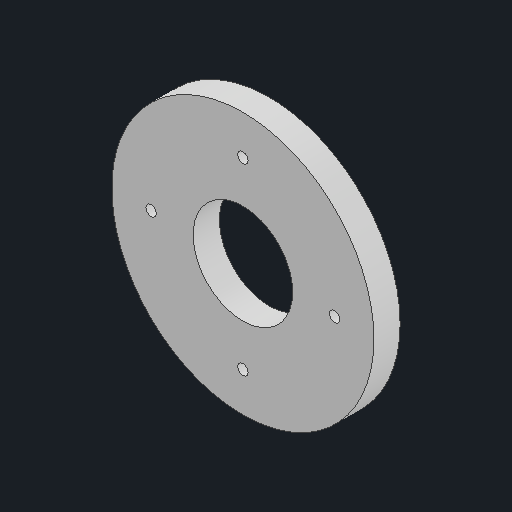
# Autodesk Inventor part: drive sprocket flange
Saved by Autodesk Inventor 2023.2 (Build 272271030, 271C)
## iProperties
Created: 2023-04-05
Part Number: drive sprocket flange
Material: Generic
Document SubType Name: Modeling
Designer: ralph
Density: 1 g/cm^3
Appearance: Default
Author: ralph
Autodesk Inventor part; units mm, degrees
ref_plane "YZ Plane" through (0, 0, 0) normal (1, 0, 0) x (0, 1, 0)
ref_plane "XZ Plane" through (0, 0, 0) normal (0, 1, 0) x (-1, 0, 0)
ref_plane "XY Plane" through (0, 0, 0) normal (0, 0, 1) x (1, 0, 0)
sketch "Sketch1" plane through (0, 0, 0) normal (0, 0, 1) x (1, 0, 0)
  arc A0 (9.4191, 43.3754) -> (11.0761, 45.5644) centre (1.4765, 51.109) ccw projected
  arc A1 (2.6827, 44.1627) -> (9.4191, 43.3754) centre (6.35, 46.3277) ccw projected
  arc A2 (1.5753, 46.6749) -> (2.6827, 44.1627) centre (12.1948, 49.8562) ccw projected
  arc A3 (-9.4191, 43.3754) -> (-2.6827, 44.1627) centre (-6.35, 46.3277) ccw projected
  arc A4 (-11.0761, 45.5644) -> (-9.4191, 43.3754) centre (-1.4765, 51.109) ccw projected
  arc A5 (-21.0132, 39.8183) -> (-14.64, 42.138) centre (-18.7077, 43.3989) ccw projected
  arc A6 (-23.1303, 41.5662) -> (-21.0132, 39.8183) centre (-15.0682, 49.1752) ccw projected
  arc A7 (-31.4745, 33.6834) -> (-25.808, 37.4103) centre (-30.0568, 37.6992) ccw projected
  arc A8 (-33.9376, 34.896) -> (-31.4745, 33.6834) centre (-27.8475, 44.1591) ccw projected
  arc A9 (-40.2389, 25.3013) -> (-35.5847, 30.2346) centre (-39.7856, 29.5357) ccw projected
  arc A10 (-42.9153, 25.9131) -> (-40.2389, 25.3013) centre (-39.1256, 36.331) ccw projected
  arc A11 (-46.8341, 15.1239) -> (-43.443, 20.9975) centre (-47.3695, 19.3488) ccw projected
  arc A12 (-49.5794, 15.1021) -> (-46.8341, 15.1239) centre (-48.2944, 26.1131) ccw projected
  arc A13 (-50.9044, 3.6999) -> (-48.9593, 10.1973) centre (-52.3997, 7.6874) ccw projected
  arc A14 (-53.5707, 3.0455) -> (-50.9044, 3.6999) centre (-54.8597, 14.0561) ccw projected
  arc A15 (-52.2305, -8.3548) -> (-51.8361, -1.584) centre (-54.605, -4.8196) ccw projected
  arc A16 (-54.674, -9.6064) -> (-52.2305, -8.3548) centre (-58.4674, 0.8101) ccw projected
  arc A17 (-50.7408, -20.3904) -> (-51.9185, -13.7112) centre (-53.8666, -17.4981) ccw projected
  arc A18 (-52.8298, -22.1718) -> (-50.7408, -20.3904) centre (-58.9232, -12.9109) ccw projected
  arc A19 (-46.5156, -31.7581) -> (-49.2019, -25.5305) centre (-50.2242, -29.6646) ccw projected
  arc A20 (-48.1375, -33.9732) -> (-46.5156, -31.7581) centre (-56.2023, -26.3671) ccw projected
  arc A21 (-39.7828, -41.8449) -> (-43.8329, -36.4047) centre (-43.8742, -40.6631) ccw projected
  arc A22 (-40.8501, -44.3744) -> (-39.7828, -41.8449) centre (-50.4517, -38.8332) ccw projected
  arc A23 (-30.9053, -50.1072) -> (-36.1008, -45.7476) centre (-35.1589, -49.9008) ccw projected
  arc A24 (-31.3605, -52.8146) -> (-30.9053, -50.1072) centre (-41.9811, -49.637) ccw projected
  arc A25 (-20.3617, -56.0994) -> (-26.4225, -53.0555) centre (-24.5482, -56.8795) ccw projected
  arc A26 (-20.1802, -58.8388) -> (-20.3617, -56.0994) centre (-31.2473, -58.1962) ccw projected
  arc A27 (-8.7203, -59.4986) -> (-15.3198, -57.9345) centre (-12.6141, -61.2232) ccw projected
  arc A28 (-7.912, -62.1223) -> (-8.7203, -59.4986) centre (-18.829, -64.0493) ccw projected
  arc A29 (3.3911, -60.1215) -> (-3.3911, -60.1215) centre (0, -62.6976) ccw projected
  arc A30 (4.7827, -62.4881) -> (3.3911, -60.1215) centre (-5.3956, -66.8807) ccw projected
  arc A31 (15.3198, -57.9345) -> (8.7203, -59.4986) centre (12.6141, -61.2232) ccw projected
  arc A32 (17.2196, -59.9164) -> (15.3198, -57.9345) centre (8.3287, -66.5379) ccw projected
  arc A33 (26.4225, -53.0555) -> (20.3617, -56.0994) centre (24.5482, -56.8795) ccw projected
  arc A34 (28.7282, -54.5458) -> (26.4225, -53.0555) centre (21.6039, -63.0393) ccw projected
  arc A35 (36.1008, -45.7476) -> (30.9053, -50.1072) centre (35.1589, -49.9008) ccw projected
  arc A36 (38.688, -46.666) -> (36.1008, -45.7476) centre (33.7145, -56.5735) ccw projected
  arc A37 (43.8329, -36.4047) -> (39.7828, -41.8449) centre (43.8742, -40.6631) ccw projected
  arc A38 (46.5622, -36.7017) -> (43.8329, -36.4047) centre (44.0076, -47.4891) ccw projected
  arc A39 (49.2019, -25.5305) -> (46.5156, -31.7581) centre (50.2242, -29.6646) ccw projected
  arc A40 (51.9262, -25.19) -> (49.2019, -25.5305) centre (51.9282, -36.2758) ccw projected
  arc A41 (51.9185, -13.7112) -> (50.7408, -20.3904) centre (53.8666, -17.4981) ccw projected
  arc A42 (54.4908, -12.7517) -> (51.9185, -13.7112) centre (57.0493, -23.5382) ccw projected
  arc A43 (51.8361, -1.584) -> (52.2305, -8.3548) centre (54.605, -4.8196) ccw projected
  arc A44 (54.1178, -0.0572) -> (51.8361, -1.584) centre (59.0949, -9.9629) ccw projected
  arc A45 (48.9593, 10.1973) -> (50.9044, 3.6999) centre (52.3997, 7.6874) ccw projected
  arc A46 (50.8273, 12.2092) -> (48.9593, 10.1973) centre (57.9546, 3.7182) ccw projected
  arc A47 (43.443, 20.9975) -> (46.8341, 15.1239) centre (47.3695, 19.3488) ccw projected
  arc A48 (44.7967, 23.386) -> (43.443, 20.9975) centre (53.69, 16.7676) ccw projected
  arc A49 (35.5847, 30.2346) -> (40.2389, 25.3013) centre (39.7856, 29.5357) ccw projected
  arc A50 (36.3511, 32.8708) -> (35.5847, 30.2346) centre (46.531, 28.4818) ccw projected
  arc A51 (25.808, 37.4103) -> (31.4745, 33.6834) centre (30.0568, 37.6992) ccw projected
  arc A52 (25.9458, 40.1523) -> (25.808, 37.4103) centre (36.8635, 38.2292) ccw projected
  arc A53 (14.64, 42.138) -> (21.0132, 39.8183) centre (18.7077, 43.3989) ccw projected
  arc A54 (14.1417, 44.8378) -> (14.64, 42.138) centre (25.2086, 45.4844) ccw projected
  circle A55 centre (0, -8) radius 12.065
  circle A56 centre (0, -8) radius 22.225
  circle A57 centre (0, -8) radius 31.75
  circle A58 centre (22.225, -8) radius 1.27
  circle A59 centre (0, -30.225) radius 1.27
  circle A60 centre (-22.225, -8) radius 1.27
  circle A61 centre (0, 14.225) radius 1.27
  circle A62 centre (0, -8) radius 12.065 projected
  ellipse E0 centre (12.8803, 49.8016) end of major axis (24.6386, 49.2708) minor radius 11.3649 (1.4863, 46.9888) -> (1.5753, 46.6749) ccw projected
  line L0 (1.4863, 46.9888) -> (1.1981, 48.0928) projected
  arc A63 (1.1981, 48.0928) -> (0.2767, 50.1653) centre (-5.564, 46.3277) ccw projected
  arc A64 (0.2767, 50.1653) -> (-0.2767, 50.1653) centre (0, -8) ccw projected
  arc A65 (-0.2767, 50.1653) -> (-1.1981, 48.0928) centre (5.564, 46.3277) ccw projected
  line L1 (-1.1981, 48.0928) -> (-1.4863, 46.9888) projected
  arc A66 (-2.6827, 44.1627) -> (-1.5753, 46.6749) centre (-12.1948, 49.8562) ccw projected
  ellipse E1 centre (-0.7968, 51.214) end of major axis (10.7669, 53.4091) minor radius 11.3649 (-11.2351, 45.8493) -> (-11.0761, 45.5644) ccw projected
  line L2 (-11.2351, 45.8493) -> (-11.7701, 46.8571) projected
  arc A67 (-11.7701, 46.8571) -> (-13.1446, 48.6613) centre (-17.9429, 43.5802) ccw projected
  arc A68 (-13.1446, 48.6613) -> (-13.6831, 48.5337) centre (0, -8) ccw projected
  arc A69 (-13.6831, 48.5337) -> (-14.1017, 46.3046) centre (-7.1148, 46.1465) ccw projected
  line L3 (-14.1017, 46.3046) -> (-14.1275, 45.1638) projected
  arc A70 (-14.64, 42.138) -> (-14.1417, 44.8378) centre (-25.2086, 45.4844) ccw projected
  ellipse E2 centre (-14.431, 49.4341) end of major axis (-3.6852, 54.2369) minor radius 11.3649 (-23.3508, 41.8068) -> (-23.1303, 41.5662) ccw projected
  line L4 (-23.3508, 41.8068) -> (-24.1038, 42.6641) projected
  arc A71 (-24.1038, 42.6641) -> (-25.8573, 44.1026) centre (-29.3544, 38.0519) ccw projected
  arc A72 (-25.8573, 44.1026) -> (-26.3518, 43.8543) centre (0, -8) ccw projected
  arc A73 (-26.3518, 43.8543) -> (-26.2451, 41.5887) centre (-19.4101, 43.0461) ccw projected
  line L5 (-26.2451, 41.5887) -> (-26.0071, 40.4728) projected
  arc A74 (-25.808, 37.4103) -> (-25.9458, 40.1523) centre (-36.8635, 38.2292) ccw projected
  ellipse E3 centre (-27.2872, 44.5579) end of major axis (-17.9387, 51.7094) minor radius 11.3649 (-34.2076, 35.0792) -> (-33.9376, 34.896) ccw projected
  line L6 (-34.2076, 35.0792) -> (-35.138, 35.7397) projected
  arc A75 (-35.138, 35.7397) -> (-37.176, 36.7351) centre (-39.1835, 30.041) ccw projected
  arc A76 (-37.176, 36.7351) -> (-37.5999, 36.3794) centre (0, -8) ccw projected
  arc A77 (-37.5999, 36.3794) -> (-36.9736, 34.1995) centre (-30.6589, 37.1939) ccw projected
  line L7 (-36.9736, 34.1995) -> (-36.4847, 33.1685) projected
  arc A78 (-35.5847, 30.2346) -> (-36.3511, 32.8708) centre (-46.531, 28.4818) ccw projected
  ellipse E4 centre (-38.6724, 36.8483) end of major axis (-31.2251, 45.963) minor radius 11.3649 (-43.2203, 26.0292) -> (-42.9153, 25.9131) ccw projected
  line L8 (-43.2203, 26.0292) -> (-44.2779, 26.4573) projected
  arc A79 (-44.2779, 26.4573) -> (-46.4905, 26.9559) centre (-46.9001, 19.9793) ccw projected
  arc A80 (-46.4905, 26.9559) -> (-46.821, 26.512) centre (0, -8) ccw projected
  arc A81 (-46.821, 26.512) -> (-45.7088, 24.5353) centre (-40.2549, 28.9053) ccw projected
  line L9 (-45.7088, 24.5353) -> (-44.9953, 23.6449) projected
  arc A82 (-43.443, 20.9975) -> (-44.7967, 23.386) centre (-53.69, 16.7676) ccw projected
  ellipse E5 centre (-47.9727, 26.721) end of major axis (-42.8281, 37.3074) minor radius 11.3649 (-49.9029, 15.1447) -> (-49.5794, 15.1021) ccw projected
  line L10 (-49.9029, 15.1447) -> (-51.0308, 15.3173) projected
  arc A83 (-51.0308, 15.3173) -> (-53.2988, 15.2922) centre (-52.0884, 8.4092) ccw projected
  arc A84 (-53.2988, 15.2922) -> (-53.518, 14.784) centre (0, -8) ccw projected
  arc A85 (-53.518, 14.784) -> (-51.9799, 13.1172) centre (-47.6808, 18.6271) ccw projected
  line L11 (-51.9799, 13.1172) -> (-51.0803, 12.4152) projected
  arc A86 (-48.9593, 10.1973) -> (-50.8273, 12.2092) centre (-57.9546, 3.7182) ccw projected
  ellipse E6 centre (-54.6868, 14.7218) end of major axis (-52.1223, 26.2093) minor radius 11.3649 (-53.8953, 3.0124) -> (-53.5707, 3.0455) ccw projected
  line L12 (-53.8953, 3.0124) -> (-55.0326, 2.9203) projected
  arc A87 (-55.0326, 2.9203) -> (-57.2336, 2.3728) centre (-54.4685, -4.0456) ccw projected
  arc A88 (-57.2336, 2.3728) -> (-57.3297, 1.8278) centre (0, -8) ccw projected
  arc A89 (-57.3297, 1.8278) -> (-55.4487, 0.5606) centre (-52.5362, 6.9134) ccw projected
  line L13 (-55.4487, 0.5606) -> (-54.4115, 0.085) projected
  arc A90 (-51.8361, -1.584) -> (-54.1178, -0.0572) centre (-59.0949, -9.9629) ccw projected
  ellipse E7 centre (-58.4527, 1.4977) end of major axis (-58.6065, 13.2669) minor radius 11.3649 (-54.9822, -9.7136) -> (-54.674, -9.6064) ccw projected
  line L14 (-54.9822, -9.7136) -> (-56.0676, -10.0655) projected
  arc A91 (-56.0676, -10.0655) -> (-58.083, -11.1058) centre (-53.9123, -16.7135) ccw projected
  arc A92 (-58.083, -11.1058) -> (-58.0508, -11.6583) centre (0, -8) ccw projected
  arc A93 (-58.0508, -11.6583) -> (-55.9283, -12.4575) centre (-54.5593, -5.6043) ccw projected
  line L15 (-55.9283, -12.4575) -> (-54.8093, -12.6811) projected
  arc A94 (-51.9185, -13.7112) -> (-54.4908, -12.7517) centre (-57.0493, -23.5382) ccw projected
  ellipse E8 centre (-59.0674, -12.2385) end of major axis (-61.9313, -0.8219) minor radius 11.3649 (-53.105, -22.3471) -> (-52.8298, -22.1718) ccw projected
  line L16 (-53.105, -22.3471) -> (-54.08, -22.9399) projected
  arc A95 (-54.08, -22.9399) -> (-55.8011, -24.4169) centre (-50.4496, -28.9116) ccw projected
  arc A96 (-55.8011, -24.4169) -> (-55.6424, -24.9471) centre (0, -8) ccw projected
  arc A97 (-55.6424, -24.9471) -> (-53.3927, -25.2353) centre (-53.6412, -18.2511) ccw projected
  line L17 (-53.3927, -25.2353) -> (-52.2524, -25.1948) projected
  arc A98 (-49.2019, -25.5305) -> (-51.9262, -25.19) centre (-51.9282, -36.2758) ccw projected
  ellipse E9 centre (-56.4978, -25.7461) end of major axis (-61.9173, -15.2977) minor radius 11.3649 (-48.3648, -34.2073) -> (-48.1375, -33.9732) ccw projected
  line L18 (-48.3648, -34.2073) -> (-49.1769, -35.0089) projected
  arc A99 (-49.1769, -35.0089) -> (-50.511, -36.843) centre (-44.2672, -39.9824) ccw projected
  arc A100 (-50.511, -36.843) -> (-50.2343, -37.3223) centre (0, -8) ccw projected
  arc A101 (-50.2343, -37.3223) -> (-47.9788, -37.084) centre (-49.8312, -30.3453) ccw projected
  line L19 (-47.9788, -37.084) -> (-46.8786, -36.7815) projected
  arc A102 (-43.8329, -36.4047) -> (-46.5622, -36.7017) centre (-44.0076, -47.4891) ccw projected
  ellipse E10 centre (-50.8824, -38.297) end of major axis (-58.5653, -29.3801) minor radius 11.3649 (-41.0173, -44.6545) -> (-40.8501, -44.3744) ccw projected
  line L20 (-41.0173, -44.6545) -> (-41.6226, -45.6218) projected
  arc A103 (-41.6226, -45.6218) -> (-42.4978, -47.7142) centre (-35.6983, -49.3291) ccw projected
  arc A104 (-42.4978, -47.7142) -> (-42.118, -48.1167) centre (0, -8) ccw projected
  arc A105 (-42.118, -48.1167) -> (-39.9783, -47.3647) centre (-43.3348, -41.2348) ccw projected
  line L21 (-39.9783, -47.3647) -> (-38.9775, -46.8167) projected
  arc A106 (-36.1008, -45.7476) -> (-38.688, -46.666) centre (-33.7145, -56.5735) ccw projected
  ellipse E11 centre (-42.5239, -49.2147) end of major axis (-52.0561, -42.3099) minor radius 11.3649 (-31.4586, -53.1258) -> (-31.3605, -52.8146) ccw projected
  line L22 (-31.4586, -53.1258) -> (-31.8245, -54.2065) projected
  arc A107 (-31.8245, -54.2065) -> (-32.1936, -56.4444) centre (-25.2049, -56.4476) ccw projected
  arc A108 (-32.1936, -56.4444) -> (-31.7312, -56.7485) centre (0, -8) ccw projected
  arc A109 (-31.7312, -56.7485) -> (-29.8226, -55.5232) centre (-34.5022, -50.3327) ccw projected
  line L23 (-29.8226, -55.5232) -> (-28.9751, -54.7592) projected
  arc A110 (-26.4225, -53.0555) -> (-28.7282, -54.5458) centre (-21.6039, -63.0393) ccw projected
  ellipse E12 centre (-31.8729, -57.9104) end of major axis (-42.7405, -53.3901) minor radius 11.3649 (-20.2039, -59.1642) -> (-20.1802, -58.8388) ccw projected
  line L24 (-20.2039, -59.1642) -> (-20.3107, -60.3003) projected
  arc A111 (-20.3107, -60.3003) -> (-20.1537, -62.5629) centre (-13.3527, -60.9544) ccw projected
  arc A112 (-20.1537, -62.5629) -> (-19.6337, -62.7522) centre (0, -8) ccw projected
  arc A113 (-19.6337, -62.7522) -> (-18.0591, -61.1198) centre (-23.8096, -57.1484) ccw projected
  line L25 (-18.0591, -61.1198) -> (-17.4107, -60.1809) projected
  arc A114 (-15.3198, -57.9345) -> (-17.2196, -59.9164) centre (-8.3287, -66.5379) ccw projected
  ellipse E13 centre (-19.5036, -63.9154) end of major axis (-31.1208, -62.0232) minor radius 11.3649 (-7.86, -62.4444) -> (-7.912, -62.1223) ccw projected
  line L26 (-7.86, -62.4444) -> (-7.7019, -63.5745) projected
  arc A115 (-7.7019, -63.5745) -> (-7.0274, -65.7399) centre (-0.7807, -62.6063) ccw projected
  arc A116 (-7.0274, -65.7399) -> (-6.4777, -65.8042) centre (0, -8) ccw projected
  arc A117 (-6.4777, -65.8042) -> (-5.322, -63.8527) centre (-11.8334, -61.3144) ccw projected
  line L27 (-5.322, -63.8527) -> (-4.9076, -62.7895) projected
  arc A118 (-3.3911, -60.1215) -> (-4.7827, -62.4881) centre (5.3956, -66.8807) ccw projected
  ellipse E14 centre (-6.0829, -66.9061) end of major axis (-17.8233, -67.7439) minor radius 11.3649 (4.9076, -62.7895) -> (4.7827, -62.4881) ccw projected
  line L28 (4.9076, -62.7895) -> (5.322, -63.8527) projected
  arc A119 (5.322, -63.8527) -> (6.4777, -65.8042) centre (11.8334, -61.3144) ccw projected
  arc A120 (6.4777, -65.8042) -> (7.0274, -65.7399) centre (0, -8) ccw projected
  arc A121 (7.0274, -65.7399) -> (7.7019, -63.5745) centre (0.7807, -62.6063) ccw projected
  line L29 (7.7019, -63.5745) -> (7.86, -62.4444) projected
  arc A122 (8.7203, -59.4986) -> (7.912, -62.1223) centre (18.829, -64.0493) ccw projected
  ellipse E15 centre (7.6657, -66.7211) end of major axis (-3.565, -70.2439) minor radius 11.3649 (17.4107, -60.1809) -> (17.2196, -59.9164) ccw projected
  line L30 (17.4107, -60.1809) -> (18.0591, -61.1198) projected
  arc A123 (18.0591, -61.1198) -> (19.6337, -62.7522) centre (23.8096, -57.1484) ccw projected
  arc A124 (19.6337, -62.7522) -> (20.1537, -62.5629) centre (0, -8) ccw projected
  arc A125 (20.1537, -62.5629) -> (20.3107, -60.3003) centre (13.3527, -60.9544) ccw projected
  line L31 (20.3107, -60.3003) -> (20.2039, -59.1642) projected
  arc A126 (20.3617, -56.0994) -> (20.1802, -58.8388) centre (31.2473, -58.1962) ccw projected
  ellipse E16 centre (21.0011, -63.3704) end of major axis (10.8856, -69.3882) minor radius 11.3649 (28.9751, -54.7592) -> (28.7282, -54.5458) ccw projected
  line L32 (28.9751, -54.7592) -> (29.8226, -55.5232) projected
  arc A127 (29.8226, -55.5232) -> (31.7312, -56.7485) centre (34.5022, -50.3327) ccw projected
  arc A128 (31.7312, -56.7485) -> (32.1936, -56.4444) centre (0, -8) ccw projected
  arc A129 (32.1936, -56.4444) -> (31.8245, -54.2065) centre (25.2049, -56.4476) ccw projected
  line L33 (31.8245, -54.2065) -> (31.4586, -53.1258) projected
  arc A130 (30.9053, -50.1072) -> (31.3605, -52.8146) centre (41.9811, -49.637) ccw projected
  ellipse E17 centre (33.2043, -57.0347) end of major axis (24.7492, -65.2231) minor radius 11.3649 (38.9775, -46.8167) -> (38.688, -46.666) ccw projected
  line L34 (38.9775, -46.8167) -> (39.9783, -47.3647) projected
  arc A131 (39.9783, -47.3647) -> (42.118, -48.1167) centre (43.3348, -41.2348) ccw projected
  arc A132 (42.118, -48.1167) -> (42.4978, -47.7142) centre (0, -8) ccw projected
  arc A133 (42.4978, -47.7142) -> (41.6226, -45.6218) centre (35.6983, -49.3291) ccw projected
  line L35 (41.6226, -45.6218) -> (41.0173, -44.6545) projected
  arc A134 (39.7828, -41.8449) -> (40.8501, -44.3744) centre (50.4517, -38.8332) ccw projected
  ellipse E18 centre (43.6175, -48.0555) end of major axis (37.2787, -57.9731) minor radius 11.3649 (46.8786, -36.7815) -> (46.5622, -36.7017) ccw projected
  line L36 (46.8786, -36.7815) -> (47.9788, -37.084) projected
  arc A135 (47.9788, -37.084) -> (50.2343, -37.3223) centre (49.8312, -30.3453) ccw projected
  arc A136 (50.2343, -37.3223) -> (50.511, -36.843) centre (0, -8) ccw projected
  arc A137 (50.511, -36.843) -> (49.1769, -35.0089) centre (44.2672, -39.9824) ccw projected
  line L37 (49.1769, -35.0089) -> (48.3648, -34.2073) projected
  arc A138 (46.5156, -31.7581) -> (48.1375, -33.9732) centre (56.2023, -26.3671) ccw projected
  ellipse E19 centre (51.6792, -36.9169) end of major axis (47.7984, -48.029) minor radius 11.3649 (52.2524, -25.1948) -> (51.9262, -25.19) ccw projected
  line L38 (52.2524, -25.1948) -> (53.3927, -25.2353) projected
  arc A139 (53.3927, -25.2353) -> (55.6424, -24.9471) centre (53.6412, -18.2511) ccw projected
  arc A140 (55.6424, -24.9471) -> (55.8011, -24.4169) centre (0, -8) ccw projected
  arc A141 (55.8011, -24.4169) -> (54.08, -22.9399) centre (50.4496, -28.9116) ccw projected
  line L39 (54.08, -22.9399) -> (53.105, -22.3471) projected
  arc A142 (50.7408, -20.3904) -> (52.8298, -22.1718) centre (58.9232, -12.9109) ccw projected
  ellipse E20 centre (56.9549, -24.2194) end of major axis (55.7413, -35.9269) minor radius 11.3649 (54.8093, -12.6811) -> (54.4908, -12.7517) ccw projected
  line L40 (54.8093, -12.6811) -> (55.9283, -12.4575) projected
  arc A143 (55.9283, -12.4575) -> (58.0508, -11.6583) centre (54.5593, -5.6043) ccw projected
  arc A144 (58.0508, -11.6583) -> (58.083, -11.1058) centre (0, -8) ccw projected
  arc A145 (58.083, -11.1058) -> (56.0676, -10.0655) centre (53.9123, -16.7135) ccw projected
  line L41 (56.0676, -10.0655) -> (54.9822, -9.7136) projected
  arc A146 (52.2305, -8.3548) -> (54.674, -9.6064) centre (58.4674, 0.8101) ccw projected
  ellipse E21 centre (59.1601, -10.6475) end of major axis (60.6792, -22.3193) minor radius 11.3649 (54.4115, 0.085) -> (54.1178, -0.0572) ccw projected
  line L42 (54.4115, 0.085) -> (55.4487, 0.5606) projected
  arc A147 (55.4487, 0.5606) -> (57.3297, 1.8278) centre (52.5362, 6.9134) ccw projected
  arc A148 (57.3297, 1.8278) -> (57.2336, 2.3728) centre (0, -8) ccw projected
  arc A149 (57.2336, 2.3728) -> (55.0326, 2.9203) centre (54.4685, -4.0456) ccw projected
  line L43 (55.0326, 2.9203) -> (53.8953, 3.0124) projected
  arc A150 (50.9044, 3.6999) -> (53.5707, 3.0455) centre (54.8597, 14.0561) ccw projected
  ellipse E22 centre (58.176, 3.0671) end of major axis (62.3459, -7.9398) minor radius 11.3649 (51.0803, 12.4152) -> (50.8273, 12.2092) ccw projected
  line L44 (51.0803, 12.4152) -> (51.9799, 13.1172) projected
  arc A151 (51.9799, 13.1172) -> (53.518, 14.784) centre (47.6808, 18.6271) ccw projected
  arc A152 (53.518, 14.784) -> (53.2988, 15.2922) centre (0, -8) ccw projected
  arc A153 (53.2988, 15.2922) -> (51.0308, 15.3173) centre (52.0884, 8.4092) ccw projected
  line L45 (51.0308, 15.3173) -> (49.9029, 15.1447) projected
  arc A154 (46.8341, 15.1239) -> (49.5794, 15.1021) centre (48.2944, 26.1131) ccw projected
  ellipse E23 centre (54.0556, 16.1851) end of major axis (60.6514, 6.4366) minor radius 11.3649 (44.9953, 23.6449) -> (44.7967, 23.386) ccw projected
  line L46 (44.9953, 23.6449) -> (45.7088, 24.5353) projected
  arc A155 (45.7088, 24.5353) -> (46.821, 26.512) centre (40.2549, 28.9053) ccw projected
  arc A156 (46.821, 26.512) -> (46.4905, 26.9559) centre (0, -8) ccw projected
  arc A157 (46.4905, 26.9559) -> (44.2779, 26.4573) centre (46.9001, 19.9793) ccw projected
  line L47 (44.2779, 26.4573) -> (43.2203, 26.0292) projected
  arc A158 (40.2389, 25.3013) -> (42.9153, 25.9131) centre (39.1256, 36.331) ccw projected
  ellipse E24 centre (47.0211, 27.9993) end of major axis (55.6873, 20.0346) minor radius 11.3649 (36.4847, 33.1685) -> (36.3511, 32.8708) ccw projected
  line L48 (36.4847, 33.1685) -> (36.9736, 34.1995) projected
  arc A159 (36.9736, 34.1995) -> (37.5999, 36.3794) centre (30.6589, 37.1939) ccw projected
  arc A160 (37.5999, 36.3794) -> (37.176, 36.7351) centre (0, -8) ccw projected
  arc A161 (37.176, 36.7351) -> (35.138, 35.7397) centre (39.1835, 30.041) ccw projected
  line L49 (35.138, 35.7397) -> (34.2076, 35.0792) projected
  arc A162 (31.4745, 33.6834) -> (33.9376, 34.896) centre (27.8475, 44.1591) ccw projected
  ellipse E25 centre (37.4516, 37.8727) end of major axis (47.721, 32.1213) minor radius 11.3649 (26.0071, 40.4728) -> (25.9458, 40.1523) ccw projected
  line L50 (26.0071, 40.4728) -> (26.2451, 41.5887) projected
  arc A163 (26.2451, 41.5887) -> (26.3518, 43.8543) centre (19.4101, 43.0461) ccw projected
  arc A164 (26.3518, 43.8543) -> (25.8573, 44.1026) centre (0, -8) ccw projected
  arc A165 (25.8573, 44.1026) -> (24.1038, 42.6641) centre (29.3544, 38.0519) ccw projected
  line L51 (24.1038, 42.6641) -> (23.3508, 41.8068) projected
  arc A166 (21.0132, 39.8183) -> (23.1303, 41.5662) centre (15.0682, 49.1752) ccw projected
  ellipse E26 centre (25.8631, 45.2731) end of major axis (37.1821, 42.045) minor radius 11.3649 (14.1275, 45.1638) -> (14.1417, 44.8378) ccw projected
  line L52 (14.1275, 45.1638) -> (14.1017, 46.3046) projected
  arc A167 (14.1017, 46.3046) -> (13.6831, 48.5337) centre (7.1148, 46.1465) ccw projected
  arc A168 (13.6831, 48.5337) -> (13.1446, 48.6613) centre (0, -8) ccw projected
  arc A169 (13.1446, 48.6613) -> (11.7701, 46.8571) centre (17.9429, 43.5802) ccw projected
  line L53 (11.7701, 46.8571) -> (11.2351, 45.8493) projected
  ellipse E27 centre (0.7968, 51.214) end of major axis (-10.7669, 53.4091) minor radius 11.3649 (11.0761, 45.5644) -> (11.2351, 45.8493) ccw projected
  circle A170 centre (22.225, -8) radius 2.3812 projected
  circle A171 centre (0, 14.225) radius 2.3812 projected
  circle A172 centre (0, -30.225) radius 2.3812 projected
  circle A173 centre (-22.225, -8) radius 2.3812 projected
  ellipse E28 centre (-12.8803, 49.8016) end of major axis (-24.6386, 49.2708) minor radius 11.3649 (-1.5753, 46.6749) -> (-1.4863, 46.9888) ccw projected
  ellipse E29 centre (-25.8631, 45.2731) end of major axis (-37.1821, 42.045) minor radius 11.3649 (-14.1417, 44.8378) -> (-14.1275, 45.1638) ccw projected
  ellipse E30 centre (-37.4516, 37.8727) end of major axis (-47.721, 32.1213) minor radius 11.3649 (-25.9458, 40.1523) -> (-26.0071, 40.4728) ccw projected
  ellipse E31 centre (-47.0211, 27.9993) end of major axis (-55.6873, 20.0346) minor radius 11.3649 (-36.3511, 32.8708) -> (-36.4847, 33.1685) ccw projected
  ellipse E32 centre (-54.0556, 16.1851) end of major axis (-60.6514, 6.4366) minor radius 11.3649 (-44.7967, 23.386) -> (-44.9953, 23.6449) ccw projected
  ellipse E33 centre (-58.176, 3.0671) end of major axis (-62.3459, -7.9398) minor radius 11.3649 (-50.8273, 12.2092) -> (-51.0803, 12.4152) ccw projected
  ellipse E34 centre (-59.1601, -10.6475) end of major axis (-60.6792, -22.3193) minor radius 11.3649 (-54.1178, -0.0572) -> (-54.4115, 0.085) ccw projected
  ellipse E35 centre (-56.9549, -24.2194) end of major axis (-55.7413, -35.9269) minor radius 11.3649 (-54.4908, -12.7517) -> (-54.8093, -12.6811) ccw projected
  ellipse E36 centre (-51.6792, -36.9169) end of major axis (-47.7984, -48.029) minor radius 11.3649 (-51.9262, -25.19) -> (-52.2524, -25.1948) ccw projected
  ellipse E37 centre (-43.6175, -48.0555) end of major axis (-37.2787, -57.9731) minor radius 11.3649 (-46.5622, -36.7017) -> (-46.8786, -36.7815) ccw projected
  ellipse E38 centre (-33.2043, -57.0347) end of major axis (-24.7492, -65.2231) minor radius 11.3649 (-38.688, -46.666) -> (-38.9775, -46.8167) ccw projected
  ellipse E39 centre (-21.0011, -63.3704) end of major axis (-10.8856, -69.3882) minor radius 11.3649 (-28.7282, -54.5458) -> (-28.9751, -54.7592) ccw projected
  ellipse E40 centre (-7.6657, -66.7211) end of major axis (3.565, -70.2439) minor radius 11.3649 (-17.2196, -59.9164) -> (-17.4107, -60.1809) ccw projected
  ellipse E41 centre (6.0829, -66.9061) end of major axis (17.8233, -67.7439) minor radius 11.3649 (-4.7827, -62.4881) -> (-4.9076, -62.7895) ccw projected
  ellipse E42 centre (19.5036, -63.9154) end of major axis (31.1208, -62.0232) minor radius 11.3649 (7.912, -62.1223) -> (7.86, -62.4444) ccw projected
  ellipse E43 centre (31.8729, -57.9104) end of major axis (42.7405, -53.3901) minor radius 11.3649 (20.1802, -58.8388) -> (20.2039, -59.1642) ccw projected
  ellipse E44 centre (42.5239, -49.2147) end of major axis (52.0561, -42.3099) minor radius 11.3649 (31.3605, -52.8146) -> (31.4586, -53.1258) ccw projected
  ellipse E45 centre (50.8824, -38.297) end of major axis (58.5653, -29.3801) minor radius 11.3649 (40.8501, -44.3744) -> (41.0173, -44.6545) ccw projected
  ellipse E46 centre (56.4978, -25.7461) end of major axis (61.9173, -15.2977) minor radius 11.3649 (48.1375, -33.9732) -> (48.3648, -34.2073) ccw projected
  ellipse E47 centre (59.0674, -12.2385) end of major axis (61.9313, -0.8219) minor radius 11.3649 (52.8298, -22.1718) -> (53.105, -22.3471) ccw projected
  ellipse E48 centre (58.4527, 1.4977) end of major axis (58.6065, 13.2669) minor radius 11.3649 (54.674, -9.6064) -> (54.9822, -9.7136) ccw projected
  ellipse E49 centre (54.6868, 14.7218) end of major axis (52.1223, 26.2093) minor radius 11.3649 (53.5707, 3.0455) -> (53.8953, 3.0124) ccw projected
  ellipse E50 centre (47.9727, 26.721) end of major axis (42.8281, 37.3074) minor radius 11.3649 (49.5794, 15.1021) -> (49.9029, 15.1447) ccw projected
  ellipse E51 centre (38.6724, 36.8483) end of major axis (31.2251, 45.963) minor radius 11.3649 (42.9153, 25.9131) -> (43.2203, 26.0292) ccw projected
  ellipse E52 centre (27.2872, 44.5579) end of major axis (17.9387, 51.7094) minor radius 11.3649 (33.9376, 34.896) -> (34.2076, 35.0792) ccw projected
  ellipse E53 centre (14.431, 49.4341) end of major axis (3.6852, 54.2369) minor radius 11.3649 (23.1303, 41.5662) -> (23.3508, 41.8068) ccw projected
  point P0 (0, 0)
  dimension "d0" = 24.13
  dimension "d1" = 44.45
  dimension "d2" = 63.5
  dimension "d3" = 2.54
  dimension "d4" = 2.54
  dimension "d5" = 2.54
  dimension "d6" = 2.54
  constraints: 7 centre point, 4 point on circle, 2 coincident, 54 other
  measures "d0" diameter of A55
  measures "d1" diameter of A56
  measures "d2" diameter of A57
  measures "d3" diameter of A58
  measures "d4" diameter of A59
  measures "d5" diameter of A60
  measures "d6" diameter of A61
extrude "Extrusion1" add sketch "Sketch1" along normal blind 6.35 contours A58 A56 A170 | A56 A170 A58 | A170 A56 A172 A173 A171 | A171 A56 A61 | A56 A61 A171 | A172 A56 A59 | A56 A59 A172 | A173 A56 A60 | A56 A60 A173 | A57
body "Solid1"
